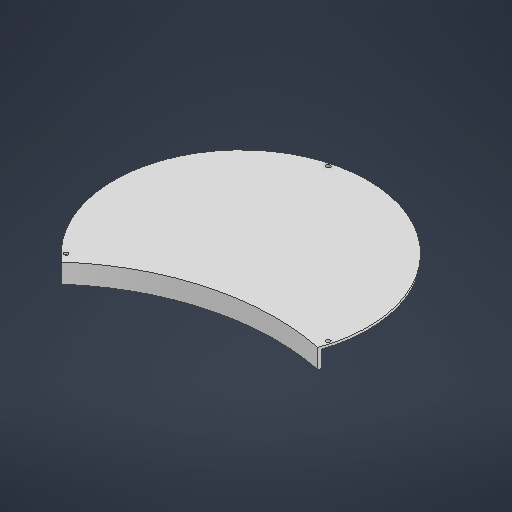
# Autodesk Inventor part: bottom_replacement_housing_bottom
Saved by Autodesk Inventor 2026 (Build 300175000, 175)
## iProperties
Created: 2025-05-12
Part Number: bottom_replacement_housing_bottom
Material: Generic
Document SubType Name: Sheet Metal
Designer: Paul Juschitz
Density: 1 g/cm^3
Sheet Metal Rule: Default_mm
Appearance: Default
Author: Paul Juschitz
Autodesk Inventor part; units mm, degrees
ref_plane "YZ Plane" through (0, 0, 0) normal (1, 0, 0) x (0, 1, 0)
ref_plane "XZ Plane" through (0, 0, 0) normal (0, 1, 0) x (-1, 0, 0)
ref_plane "XY Plane" through (0, 0, 0) normal (0, 0, 1) x (1, 0, 0)
derived "m2m_shell_3.ipt"
sketch "Sketch1" plane through (0, 0, 0) normal (0, 1, 0) x (-1, 0, 0)
  circle A0 centre (52.2558, 52.2558) radius 1.25
  circle A1 centre (19.1269, -71.3827) radius 1.25
  circle A2 centre (-71.3827, 19.1269) radius 1.25
  line L0 (52.2558, 52.2558) -> (19.1269, -71.3827) construction
  line L1 (19.1269, -71.3827) -> (-71.3827, 19.1269) construction
  line L2 (-71.3827, 19.1269) -> (52.2558, 52.2558) construction
  line L3 (-71.3827, 19.1269) -> (35.6914, -9.5635)
  line L4 (52.2558, 52.2558) -> (-26.1279, -26.1279)
  line L5 (19.1269, -71.3827) -> (-9.5635, 35.6914)
  line L6 (0, -136.5769) -> (0, 186.0374) construction
  circle A3 centre (0, 0) radius 76
  dimension "bottom_screwhole_diameter" = 2.5
  dimension "bottom_screwhole_spacing" = 128
  dimension "bottom_screwhole_angle" = 15
  dimension "d6" = 152
  constraints: 14 end point, 4 centre point, 3 midpoint, 2 coincident, 2 equal length, 2 equal radius, 2 point on line, 1 vertical, 2 other
  measures "bottom_screwhole_diameter" diameter of A0
  measures "bottom_screwhole_spacing" distance of L0.end L1.end
  measures "bottom_screwhole_angle" angle of L6 L5
  measures "d6" diameter of A3
extrude "Extrusion1" add sketch "Sketch1" along normal blind 1.5
sketch "Sketch2" plane through (0, 1.5, 0) normal (0, 1, 0) x (1, 0, 0)
  circle A0 centre (0, 0) radius 76 construction
  arc A1 (71.5806, -25.5384) -> (-49.2214, -57.9072) centre (43.599, -162.7136) ccw
  line L0 (-76, 0) -> (76, 0) construction
  line L1 (43.599, -162.7136) -> (0, 0) construction
  circle A2 centre (-52.2558, -52.2558) radius 1.25 projected
  arc A3 (-49.2214, -57.9072) -> (71.5806, -25.5384) centre (0, 0) ccw
  dimension "bottom_cutout_radius" = 140
  dimension "bottom_cutout_angle" = 105
  dimension "bottom_cutout_clearance" = 5
  constraints: 10 point on circle, 4 end point, 2 centre point, 1 concentric, 1 horizontal, 1 line through centre
  measures "bottom_cutout_radius" radius of A1
  measures "bottom_cutout_angle" angle of L0 L1
extrude "Extrusion2" cut sketch "Sketch2" against normal through all contours A3 A1
sketch "Sketch3" plane through (0, 0, 0) normal (0, -1, 0) x (1, 0, 0)
  arc A0 (-49.2214, 57.9072) -> (71.5806, 25.5384) centre (43.599, 162.7136) ccw projected
  arc A1 (-49.2214, 57.9072) -> (71.5806, 25.5384) centre (0, 0) ccw construction
  circle A2 centre (71.3827, 19.1269) radius 1.25 construction
  circle A3 centre (-52.2558, 52.2558) radius 1.25 construction
  arc A4 (72.0748, 24.1085) -> (71.5806, 25.5384) centre (0, 0) ccw
  arc A5 (-50.3644, 56.916) -> (72.0748, 24.1085) centre (43.599, 162.7136) ccw
  arc A6 (-49.2214, 57.9072) -> (-50.3644, 56.916) centre (0, 0) ccw
  dimension "d16" = 1.5
  constraints: 8 point on circle, 3 centre point, 3 coincident
  measures "d16" radial gap between concentric circles of A5 A0
extrude "Extrusion3" add sketch "Sketch3" along normal blind 10
equation "\"bottom_screwhole_diameter\" = m2m_shell_bottom_screwhole_ID"
equation "\"d6\" = 2 * m2m_bottom_radius_lower"
equation "\"d16\" = bottom_material_thickness"
equation "\"BendRadius\" = Thickness"
equation "\"BendReliefWidth\" = Thickness"
equation "\"BendReliefDepth\" = 0.5 * Thickness"
equation "\"CornerReliefSize\" = 4 * Thickness"
equation "\"MinimumRemnant\" = 2 * Thickness"
equation "\"TransitionRadius\" = BendRadius"
equation "\"JacobiRadiusSize\" = BendRadius"
equation "\"GapSize\" = Thickness"
equation "\"m2m_shell_bottom_screwhole_ID\" = 2.5"
equation "\"m2m_bottom_radius_lower\" = 76"
equation "\"bottom_material_thickness\" = 1.5"
equation "\"Thickness\" = 0.5"
body "Solid1"
